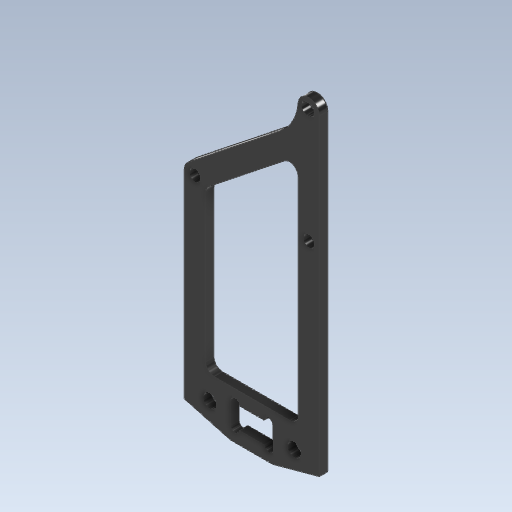
# Autodesk Inventor part: UpperArm_side_frame
Saved by Autodesk Inventor 2020.4 (Build 244396000, 396)
## iProperties
Part Number: UpperArm_side_frame
Material: GFRP
Document SubType Name: Modeling
Designer: Masato Kubotera
Density: 1.75 g/cm^3
Appearance: 低 光沢 - 黒
Description: GFRP T2
Mass: 3.2426 g
Surface Area: 26.9302 cm^2
Volume: 1.85291 cm^3
Author: Masato Kubotera
Autodesk Inventor part; units mm, degrees
ref_plane "YZ Plane" through (0, 0, 0) normal (1, 0, 0) x (0, 1, 0)
ref_plane "XZ Plane" through (0, 0, 0) normal (0, 1, 0) x (-1, 0, 0)
ref_plane "XY Plane" through (0, 0, 0) normal (0, 0, 1) x (1, 0, 0)
sketch "スケッチ1" plane through (0, 0, 0) normal (0, 0, 1) x (1, 0, 0)
  circle A0 centre (0, 0) radius 10.5 construction
  line L0 (-16, 13) -> (16, 13) construction
  line L1 (16, 13) -> (16, -30) construction
  line L2 (16, -30) -> (-16, -30) construction
  line L3 (-16, -30) -> (-16, 13) construction
  line L4 (-16, 13) -> (16, -30) construction
  line L5 (16, 13) -> (-16, -30) construction
  line L6 (0, 13) -> (0, -30) construction
  line L7 (-13.5, -28) -> (13.5, -28) construction
  line L8 (13.5, -28) -> (13.5, -1) construction
  line L9 (13.5, -1) -> (-13.5, -1) construction
  line L10 (-13.5, -1) -> (-13.5, -28) construction
  line L11 (-13.5, -28) -> (13.5, -1) construction
  line L12 (13.5, -28) -> (-13.5, -1) construction
  circle A1 centre (13.5, -28) radius 1.35
  arc A2 (13, 0.35) -> (13, -2.35) centre (13, -1) ccw
  line L13 (13, 0.35) -> (13.5, 0.35)
  line L14 (13, -2.35) -> (13.5, -2.35)
  arc A3 (13.5, -2.35) -> (13.5, 0.35) centre (13.5, -1) ccw
  circle A4 centre (-13.5, -28) radius 1.35
  line L15 (-5, -70) -> (5, -70) construction
  line L16 (5, -70) -> (5, -75) construction
  line L17 (5, -75) -> (-5, -75) construction
  line L18 (-5, -75) -> (-5, -70) construction
  line L19 (-5, -70) -> (5, -75) construction
  line L20 (5, -70) -> (-5, -75) construction
  line L21 (-5.05, -69.95) -> (-2.95, -69.95) construction
  line L22 (5.05, -69.95) -> (5.05, -75.05)
  line L23 (5.05, -75.05) -> (2.95, -75.05) construction
  line L24 (-5.05, -75.05) -> (-5.05, -69.95)
  line L25 (-5.05, -69.95) -> (5.05, -75.05) construction
  line L26 (5.05, -69.95) -> (-5.05, -75.05) construction
  arc A5 (5.05, -69.95) -> (2.95, -69.95) centre (4, -69.95) ccw
  line L27 (-5.05, -72.5) -> (5.05, -72.5) construction
  line L28 (0, -69.95) -> (0, -75.05) construction
  arc A6 (2.95, -75.05) -> (5.05, -75.05) centre (4, -75.05) ccw
  arc A7 (-2.95, -69.95) -> (-5.05, -69.95) centre (-4, -69.95) ccw
  arc A8 (-5.05, -75.05) -> (-2.95, -75.05) centre (-4, -75.05) ccw
  line L29 (-2.95, -69.95) -> (2.95, -69.95)
  line L30 (2.95, -69.95) -> (5.05, -69.95) construction
  line L31 (-2.95, -75.05) -> (-5.05, -75.05) construction
  line L32 (2.95, -75.05) -> (-2.95, -75.05)
  circle A9 centre (10, -72.5) radius 1.6
  circle A10 centre (-10, -72.5) radius 1.6
  line L33 (-5, -78) -> (5, -78)
  line L34 (5, -78) -> (16, -75)
  line L35 (16, -75) -> (16, -1)
  line L36 (-5, -78) -> (-16, -75)
  circle A11 centre (-13.5, -28) radius 2.4 construction
  arc A12 (6.8621, -8.6445) -> (11.0068, -0.8153) centre (0, 0) ccw
  line L37 (-16, -28) -> (-16, -75)
  line L38 (-15.0543, -26.0419) -> (6.8621, -8.6445)
  arc A13 (-15.0543, -26.0419) -> (-16, -28) centre (-13.5, -28) ccw
  line L39 (11, -11.7436) -> (11, -67)
  line L40 (11, -67) -> (-11, -67)
  line L41 (11, -11.7436) -> (-11, -29.2074)
  line L42 (-11, -29.2074) -> (-11, -67)
  arc A14 (16, -1) -> (11, -1) centre (13.5, -1) ccw
  point P0 (0, -8.5)
  point P1 (0, -14.5)
  point P2 (0, -72.5)
  point P3 (0, -72.5)
  dimension "d0" = 21
  dimension "d1" = 32
  dimension "d2" = 43
  dimension "d3" = 8.5
  dimension "d4" = 27
  dimension "d5" = 27
  dimension "d6" = 2.7
  dimension "d8" = 2.7
  dimension "d9" = 0.5
  dimension "d10" = 1
  dimension "d11" = 10
  dimension "d12" = 5
  dimension "d13" = 0.05
  dimension "d14" = 0.05
  dimension "d15" = 72.5
  dimension "d16" = 1.05
  dimension "d17" = 3.2
  dimension "d18" = 20
  dimension "d19" = 3
  dimension "d20" = 4.8
  dimension "d25" = 5
  dimension "d26" = 5
  dimension "d27" = 5
  dimension "d28" = 3
  constraints: 86 end point, 20 parallel, 19 point on circle, 15 centre point, 14 midpoint, 13 point on line, 10 symmetric about line, 9 tangent, 8 coincident, 7 horizontal, 7 perpendicular, 2 collinear, 1 vertical, 5 other
  measures "d0" diameter of A0
  measures "d1" distance of L1.end L2.end
  measures "d2" distance of L0.end L1.end
  measures "d3" distance of point (0, 0) point (0, -8.5)
  measures "d4" distance of L9.end L8.end
  measures "d5" distance of L8.end L7.end
  measures "d6" diameter of A1
  measures "d8" diameter of A2
  measures "d9" distance of A2.centre L8.end
  measures "d10" distance from line of L9 point (0, 0)
  measures "d11" distance of L16.end L17.end
  measures "d12" distance of L15.end L16.end
  measures "d13" distance between parallel lines of L21 L15
  measures "d14" distance between parallel lines of L22 L16
  measures "d15" distance of point (0, -72.5) point (0, 0)
  measures "d16" radius of A5
  measures "d17" diameter of A9
  measures "d18" distance of A10.centre A9.centre
  measures "d19" distance from line of L33.end L17
  measures "d20" diameter of A11
  measures "d25" distance between parallel lines of L38 L41
  measures "d26" distance between parallel lines of L39 L35
  measures "d27" distance between parallel lines of L37 L42
  measures "d28" distance between parallel lines of L15 L40
extrude "押し出し1" add sketch "スケッチ1" along normal blind 2
fillet "フィレット1" radius 2 6 edges at (11, -11.7436, 1) (11, -67, 1) (-11, -67, 1) (-11, -29.2074, 1) (-5, -78, 1) (5, -78, 1)
equation "\"d8\" = d6"
equation "\"d13\" = d14"
equation "\"d27\" = d26"
equation "\"d28\" = d19"
